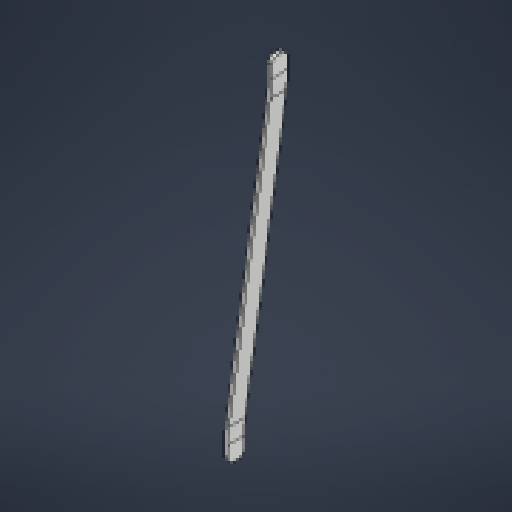
# Autodesk Inventor part: Endgame ramp polycarb
Saved by Autodesk Inventor 2023.2 (Build 272271030, 271C)
## iProperties
Created: 2023-04-06
Part Number: Endgame ramp polycarb
Material: Generic
Document SubType Name: Modeling
Designer: Main Account
Density: 1 g/cm^3
Appearance: Default
Author: Main Account
Autodesk Inventor part; units mm, degrees
ref_plane "YZ Plane" through (0, 0, 0) normal (1, 0, 0) x (0, 1, 0)
ref_plane "XZ Plane" through (0, 0, 0) normal (0, 1, 0) x (-1, 0, 0)
ref_plane "XY Plane" through (0, 0, 0) normal (0, 0, 1) x (1, 0, 0)
sketch "Sketch1" plane through (0, 0, 0) normal (0, 0, 1) x (1, 0, 0)
  line L0 (31.75, 85.8647) -> (31.75, 91.9353) construction
  line L1 (14.2875, -48.6156) -> (14.2875, -52.9844) construction
  line L2 (31.75, 93.7245) -> (31.75, 86.7628)
  line L3 (14.2875, -55.6548) -> (14.2875, -48.6931)
  line L4 (31.288, 79.9269) -> (14.7495, -41.8572)
  arc A0 (31.288, 79.9269) -> (31.75, 86.7628) centre (-19.05, 86.7628) ccw
  arc A1 (14.7495, -41.8572) -> (14.2875, -48.6931) centre (65.0875, -48.6931) ccw
  line L5 (33.3375, 93.7245) -> (33.3375, 86.7628)
  arc A2 (32.861, 79.7133) -> (33.3375, 86.7628) centre (-19.05, 86.7628) ccw
  line L6 (32.861, 79.7133) -> (16.3226, -42.0708)
  arc A3 (16.3226, -42.0708) -> (15.875, -48.6931) centre (65.0875, -48.6931) ccw
  line L7 (15.875, -48.6931) -> (15.875, -55.6548)
  line L8 (31.75, 93.7245) -> (33.3375, 93.7245)
  line L9 (14.2875, -55.6548) -> (15.875, -55.6548)
  point P0 (0, 0)
  dimension "d0" = 50.8
  dimension "d1" = 50.8
  dimension "d2" = 1.5875
  constraints: 16 end point, 8 point on circle, 4 centre point, 4 tangent, 2 point on line, 2 vertical, 1 horizontal, 1 parallel, 1 perpendicular, 4 other
  measures "d0" radius of A0
  measures "d1" radius of A1
  measures "d2" radial gap between concentric circles of A0 A2
extrude "Extrusion1" add sketch "Sketch1" against normal blind 6.35
fillet "Fillet1" radius 3.175 1 edges at (32.5437, 93.7245, 0)
fillet "Fillet2" radius 3.175 1 edges at (32.5437, 93.7245, -6.35)
fillet "Fillet3" radius 3.175 1 edges at (15.0812, -55.6548, 0)
fillet "Fillet4" radius 3.175 1 edges at (15.0812, -55.6548, -6.35)
sketch "Sketch2" plane through (33.3375, 86.7628, 0) normal (1, 0, 0) x (0, 0, -1)
  line L0 (6.35, 6.9617) -> (6.35, 0) construction
  line L1 (0, 0) -> (0, 6.9617) construction
  line L2 (0, 0) -> (6.35, 0) construction
  circle A0 centre (3.175, 3.175) radius 3.175
  point P0 (0, -86.7628)
  constraints: 3 tangent, 1 centre point
hole "Hole1" at (33.3375, 89.9378, -3.175) direction (-1, 0, 0) diameter 4.318 end through all
sketch "Sketch3" plane through (15.875, -55.6548, 0) normal (1, 0, 0) x (0, 0, -1)
  line L0 (6.35, 6.9617) -> (6.35, 0) construction
  line L1 (0, 0) -> (0, 6.9617) construction
  circle A0 centre (3.175, 3.7867) radius 3.175
  line L2 (0, 6.9617) -> (6.35, 6.9617) construction
  point P0 (0, 55.6548)
  constraints: 3 tangent, 1 centre point
hole "Hole2" at (15.875, -51.8681, -3.175) direction (-1, 0, 0) diameter 4.318 end through all
body "Solid1"
